Autodesk Inventor part; units mm, degrees
(part 2 of 2)
  line L274 (138.3563, 14.6531) -> (138.3563, 9.9031)
  line L275 (136.8563, 14.8531) -> (136.8563, 12.9031)
  line L276 (137.8563, 15.1531) -> (137.8563, 15.0531)
  line L277 (138.0563, 14.8531) -> (138.1563, 14.8531)
  line L278 (137.3563, 15.3531) -> (137.6563, 15.3531)
  line L279 (138.0563, 21.8531) -> (138.1563, 21.8531)
  line L280 (137.8563, 21.5531) -> (137.8563, 21.6531)
  line L281 (137.3563, 21.3531) -> (137.6563, 21.3531)
ref_plane "Start Plane" through (0, 0, 0) normal (0, 0, 1) x (1, 0, 0)
ref_plane "End Plane" through (0, 0, 150) normal (0, 0, 1) x (1, 0, 0)
sketch "Sketch1" plane through (0, 0, 0) normal (0, 0, 1) x (1, 0, 0)
  line L0 (-3.2324, -15.4999) -> (-0.9538, -15.4999)
  arc A0 (-0.8538, -15.5267) -> (-0.9538, -15.4999) centre (-0.9538, -15.6999) ccw
  line L1 (-0.8538, -15.5267) -> (-0.1, -15.9619)
  arc A1 (-0.1, -15.9619) -> (0.1, -15.9619) centre (0, -15.7887) ccw
  line L2 (0.1, -15.9619) -> (0.8538, -15.5267)
  arc A2 (0.9538, -15.4999) -> (0.8538, -15.5267) centre (0.9538, -15.6999) ccw
  line L3 (0.9538, -15.4999) -> (3.2324, -15.4999)
  arc A3 (3.2324, -15.4999) -> (3.586, -15.3534) centre (3.2324, -14.9999) ccw
  line L4 (3.586, -15.3534) -> (6.2929, -12.6465)
  arc A4 (6.6464, -12.5) -> (6.2929, -12.6465) centre (6.6464, -13) ccw
  line L5 (6.6464, -12.5) -> (8, -12.5)
  arc A5 (8, -12.5) -> (8.5, -12) centre (8, -12) ccw
  line L6 (8.5, -12) -> (8.5, -8)
  arc A6 (8.5, -8) -> (8, -7.5) centre (8, -8) ccw
  line L7 (8, -7.5) -> (6.6464, -7.5)
  arc A7 (6.2929, -7.3536) -> (6.6464, -7.5) centre (6.6464, -7) ccw
  line L8 (6.2929, -7.3536) -> (3.5858, -4.6465)
  arc A8 (3.5858, -4.6465) -> (3.2322, -4.5) centre (3.2322, -5) ccw
  line L9 (3.2322, -4.5) -> (0.9536, -4.5)
  arc A9 (0.8536, -4.4732) -> (0.9536, -4.5) centre (0.9536, -4.3) ccw
  line L10 (0.8536, -4.4732) -> (0.1, -4.0381)
  arc A10 (0.1, -4.0381) -> (-0.1, -4.0381) centre (0, -4.2113) ccw
  line L11 (-0.1, -4.0381) -> (-0.8536, -4.4732)
  arc A11 (5.8536, 6.9142) -> (6, 7.2678) centre (5.5, 7.2678) ccw
  line L12 (6, 8) -> (6, 7.2678)
  arc A12 (6, 8) -> (5.5, 8.5) centre (5.5, 8) ccw
  line L13 (3.5, 8.5) -> (5.5, 8.5)
  arc A13 (3, 9) -> (3.5, 8.5) centre (3.5, 9) ccw
  line L14 (3, 9.3) -> (3, 9)
  arc A14 (3.2, 9.5) -> (3, 9.3) centre (3.2, 9.3) ccw
  line L15 (3.3, 9.5) -> (3.2, 9.5)
  arc A15 (3.3, 9.5) -> (3.5, 9.7) centre (3.3, 9.7) ccw
  line L16 (3.5, 9.8) -> (3.5, 9.7)
  arc A16 (3.7, 10) -> (3.5, 9.8) centre (3.7, 9.8) ccw
  line L17 (8.5, 10) -> (3.7, 10)
  arc A17 (10, 8.5) -> (8.5, 10) centre (8.5, 8.5) ccw
  line L18 (10, 3.7) -> (10, 8.5)
  arc A18 (9.8, 3.5) -> (10, 3.7) centre (9.8, 3.7) ccw
  line L19 (9.7, 3.5) -> (9.8, 3.5)
  arc A19 (9.7, 3.5) -> (9.5, 3.3) centre (9.7, 3.3) ccw
  line L20 (9.5, 3.2) -> (9.5, 3.3)
  arc A20 (9.3, 3) -> (9.5, 3.2) centre (9.3, 3.2) ccw
  line L21 (9, 3) -> (9.3, 3)
  arc A21 (8.5, 3.5) -> (9, 3) centre (9, 3.5) ccw
  line L22 (8.5, 5.5) -> (8.5, 3.5)
  arc A22 (8.5, 5.5) -> (8, 6) centre (8, 5.5) ccw
  line L23 (7.2678, 6) -> (8, 6)
  arc A23 (7.2678, 6) -> (6.9142, 5.8536) centre (7.2678, 5.5) ccw
  line L24 (4.6464, 3.5858) -> (6.9142, 5.8536)
  arc A24 (4.6464, 3.5858) -> (4.5, 3.2322) centre (5, 3.2322) ccw
  line L25 (4.5, 0.9536) -> (4.5, 3.2322)
  arc A25 (4.4732, 0.8536) -> (4.5, 0.9536) centre (4.3, 0.9536) ccw
  line L26 (4.0381, 0.1) -> (4.4732, 0.8536)
  arc A26 (4.0381, 0.1) -> (4.0381, -0.1) centre (4.2113, 0) ccw
  line L27 (4.4732, -0.8536) -> (4.0381, -0.1)
  arc A27 (4.5, -0.9536) -> (4.4732, -0.8536) centre (4.3, -0.9536) ccw
  line L28 (4.5, -3.2322) -> (4.5, -0.9536)
  arc A28 (4.5, -3.2322) -> (4.6464, -3.5858) centre (5, -3.2322) ccw
  line L29 (6.9142, -5.8536) -> (4.6464, -3.5858)
  arc A29 (6.9142, -5.8536) -> (7.2678, -6) centre (7.2678, -5.5) ccw
  line L30 (8, -6) -> (7.2678, -6)
  arc A30 (8, -6) -> (8.5, -5.5) centre (8, -5.5) ccw
  line L31 (8.5, -3.5) -> (8.5, -5.5)
  arc A31 (9, -3) -> (8.5, -3.5) centre (9, -3.5) ccw
  line L32 (9.3, -3) -> (9, -3)
  arc A32 (9.5, -3.2) -> (9.3, -3) centre (9.3, -3.2) ccw
  line L33 (9.5, -3.3) -> (9.5, -3.2)
  arc A33 (9.5, -3.3) -> (9.7, -3.5) centre (9.7, -3.3) ccw
  line L34 (9.8, -3.5) -> (9.7, -3.5)
  arc A34 (10, -3.7) -> (9.8, -3.5) centre (9.8, -3.7) ccw
  line L35 (10, -16.35) -> (10, -3.7)
  arc A35 (9.8, -16.55) -> (10, -16.35) centre (9.8, -16.35) ccw
  line L36 (9.7, -16.55) -> (9.8, -16.55)
  arc A36 (9.7, -16.55) -> (9.5, -16.75) centre (9.7, -16.75) ccw
  line L37 (9.5, -16.85) -> (9.5, -16.75)
  arc A37 (9.3, -17.05) -> (9.5, -16.85) centre (9.3, -16.85) ccw
  line L38 (9, -17.05) -> (9.3, -17.05)
  arc A38 (8.5, -16.55) -> (9, -17.05) centre (9, -16.55) ccw
  line L39 (8.5, -14.5) -> (8.5, -16.55)
  arc A39 (8.5, -14.5) -> (8, -14) centre (8, -14.5) ccw
  line L40 (7.2678, -14) -> (8, -14)
  arc A40 (7.2678, -14) -> (6.9142, -14.1464) centre (7.2678, -14.5) ccw
  line L41 (4.6464, -16.4142) -> (6.9142, -14.1464)
  arc A41 (4.6464, -16.4142) -> (4.5, -16.7678) centre (5, -16.7678) ccw
  line L42 (4.5, -19.0464) -> (4.5, -16.7678)
  arc A42 (4.4732, -19.1464) -> (4.5, -19.0464) centre (4.3, -19.0464) ccw
  line L43 (4.0381, -19.9) -> (4.4732, -19.1464)
  arc A43 (4.0381, -19.9) -> (4.0381, -20.1) centre (4.2113, -20) ccw
  line L44 (4.4732, -20.8536) -> (4.0381, -20.1)
  arc A44 (4.5, -20.9536) -> (4.4732, -20.8536) centre (4.3, -20.9536) ccw
  line L45 (4.5, -23.2322) -> (4.5, -20.9536)
  arc A45 (4.5, -23.2322) -> (4.6464, -23.5858) centre (5, -23.2322) ccw
  line L46 (6.9142, -25.8536) -> (4.6464, -23.5858)
  arc A46 (6.9142, -25.8536) -> (7.2678, -26) centre (7.2678, -25.5) ccw
  line L47 (8, -26) -> (7.2678, -26)
  arc A47 (8, -26) -> (8.5, -25.5) centre (8, -25.5) ccw
  line L48 (8.5, -23.55) -> (8.5, -25.5)
  arc A48 (9, -23.05) -> (8.5, -23.55) centre (9, -23.55) ccw
  line L49 (9.3, -23.05) -> (9, -23.05)
  arc A49 (9.5, -23.25) -> (9.3, -23.05) centre (9.3, -23.25) ccw
  line L50 (9.5, -23.35) -> (9.5, -23.25)
  arc A50 (9.5, -23.35) -> (9.7, -23.55) centre (9.7, -23.35) ccw
  line L51 (9.8, -23.55) -> (9.7, -23.55)
  arc A51 (10, -23.75) -> (9.8, -23.55) centre (9.8, -23.75) ccw
  arc A52 (-0.9536, -4.5) -> (-0.8536, -4.4732) centre (-0.9536, -4.3) ccw
  line L52 (-0.9536, -4.5) -> (-3.2322, -4.5)
  arc A53 (-3.2322, -4.5) -> (-3.5858, -4.6465) centre (-3.2322, -5) ccw
  line L53 (-3.5858, -4.6465) -> (-6.2929, -7.3536)
  arc A54 (-6.6464, -7.5) -> (-6.2929, -7.3536) centre (-6.6464, -7) ccw
  line L54 (-6.6464, -7.5) -> (-8, -7.5)
  arc A55 (-8, -7.5) -> (-8.5, -8) centre (-8, -8) ccw
  line L55 (-8.5, -8) -> (-8.5, -12)
  arc A56 (-8.5, -12) -> (-8, -12.5) centre (-8, -12) ccw
  line L56 (-8, -12.5) -> (-6.6464, -12.5)
  arc A57 (-6.2929, -12.6465) -> (-6.6464, -12.5) centre (-6.6464, -13) ccw
  line L57 (-6.2929, -12.6465) -> (-3.586, -15.3534)
  arc A58 (-3.586, -15.3534) -> (-3.2324, -15.4999) centre (-3.2324, -14.9999) ccw
  arc A59 (-10, -28.5) -> (-8.5, -30) centre (-8.5, -28.5) ccw
  line L58 (-10, -23.75) -> (-10, -28.5)
  arc A60 (-9.8, -23.55) -> (-10, -23.75) centre (-9.8, -23.75) ccw
  line L59 (-9.7, -23.55) -> (-9.8, -23.55)
  arc A61 (-9.7, -23.55) -> (-9.5, -23.35) centre (-9.7, -23.35) ccw
  line L60 (-9.5, -23.25) -> (-9.5, -23.35)
  arc A62 (-9.3, -23.05) -> (-9.5, -23.25) centre (-9.3, -23.25) ccw
  line L61 (-9, -23.05) -> (-9.3, -23.05)
  arc A63 (-8.5, -23.55) -> (-9, -23.05) centre (-9, -23.55) ccw
  line L62 (-8.5, -25.5) -> (-8.5, -23.55)
  arc A64 (-8.5, -25.5) -> (-8, -26) centre (-8, -25.5) ccw
  line L63 (-7.2678, -26) -> (-8, -26)
  arc A65 (-7.2678, -26) -> (-6.9142, -25.8536) centre (-7.2678, -25.5) ccw
  line L64 (-4.6464, -23.5858) -> (-6.9142, -25.8536)
  arc A66 (-4.6464, -23.5858) -> (-4.5, -23.2322) centre (-5, -23.2322) ccw
  line L65 (-4.5, -20.9536) -> (-4.5, -23.2322)
  arc A67 (-4.4732, -20.8536) -> (-4.5, -20.9536) centre (-4.3, -20.9536) ccw
  line L66 (-4.0381, -20.1) -> (-4.4732, -20.8536)
  arc A68 (-4.0381, -20.1) -> (-4.0381, -19.9) centre (-4.2113, -20) ccw
  line L67 (-4.4732, -19.1464) -> (-4.0381, -19.9)
  arc A69 (-4.5, -19.0464) -> (-4.4732, -19.1464) centre (-4.3, -19.0464) ccw
  line L68 (-4.5, -16.7678) -> (-4.5, -19.0464)
  arc A70 (-4.5, -16.7678) -> (-4.6464, -16.4142) centre (-5, -16.7678) ccw
  line L69 (-6.9142, -14.1464) -> (-4.6464, -16.4142)
  arc A71 (-6.9142, -14.1464) -> (-7.2678, -14) centre (-7.2678, -14.5) ccw
  line L70 (-8, -14) -> (-7.2678, -14)
  arc A72 (-8, -14) -> (-8.5, -14.5) centre (-8, -14.5) ccw
  line L71 (-8.5, -16.55) -> (-8.5, -14.5)
  arc A73 (-9, -17.05) -> (-8.5, -16.55) centre (-9, -16.55) ccw
  line L72 (-9.3, -17.05) -> (-9, -17.05)
  arc A74 (-9.5, -16.85) -> (-9.3, -17.05) centre (-9.3, -16.85) ccw
  line L73 (-9.5, -16.75) -> (-9.5, -16.85)
  arc A75 (-9.5, -16.75) -> (-9.7, -16.55) centre (-9.7, -16.75) ccw
  line L74 (-9.8, -16.55) -> (-9.7, -16.55)
  arc A76 (-10, -16.35) -> (-9.8, -16.55) centre (-9.8, -16.35) ccw
  line L75 (-10, -3.7) -> (-10, -16.35)
  arc A77 (-9.8, -3.5) -> (-10, -3.7) centre (-9.8, -3.7) ccw
  line L76 (-9.7, -3.5) -> (-9.8, -3.5)
  arc A78 (-9.7, -3.5) -> (-9.5, -3.3) centre (-9.7, -3.3) ccw
  line L77 (-9.5, -3.2) -> (-9.5, -3.3)
  arc A79 (-9.3, -3) -> (-9.5, -3.2) centre (-9.3, -3.2) ccw
  line L78 (-9, -3) -> (-9.3, -3)
  arc A80 (-8.5, -3.5) -> (-9, -3) centre (-9, -3.5) ccw
  line L79 (-8.5, -5.45) -> (-8.5, -3.5)
  arc A81 (-8.5, -5.45) -> (-8, -5.95) centre (-8, -5.45) ccw
  line L80 (-7.2178, -5.95) -> (-8, -5.95)
  arc A82 (-7.2178, -5.95) -> (-6.8642, -5.8036) centre (-7.2178, -5.45) ccw
  line L81 (-4.6464, -3.5858) -> (-6.8642, -5.8036)
  arc A83 (-4.6464, -3.5858) -> (-4.5, -3.2322) centre (-5, -3.2322) ccw
  line L82 (-4.5, -0.9536) -> (-4.5, -3.2322)
  arc A84 (-4.4732, -0.8536) -> (-4.5, -0.9536) centre (-4.3, -0.9536) ccw
  line L83 (-4.0381, -0.1) -> (-4.4732, -0.8536)
  arc A85 (-4.0381, -0.1) -> (-4.0381, 0.1) centre (-4.2113, 0) ccw
  line L84 (-4.4732, 0.8536) -> (-4.0381, 0.1)
  arc A86 (-4.5, 0.9536) -> (-4.4732, 0.8536) centre (-4.3, 0.9536) ccw
  line L85 (-4.5, 3.2322) -> (-4.5, 0.9536)
  arc A87 (-4.5, 3.2322) -> (-4.6464, 3.5858) centre (-5, 3.2322) ccw
  line L86 (-6.9642, 5.9036) -> (-4.6464, 3.5858)
  arc A88 (-6.9642, 5.9036) -> (-7.3178, 6.05) centre (-7.3178, 5.55) ccw
  line L87 (-8, 6.05) -> (-7.3178, 6.05)
  arc A89 (-8, 6.05) -> (-8.5, 5.55) centre (-8, 5.55) ccw
  line L88 (-8.5, 3.5) -> (-8.5, 5.55)
  arc A90 (-9, 3) -> (-8.5, 3.5) centre (-9, 3.5) ccw
  line L89 (-9.3, 3) -> (-9, 3)
  arc A91 (-9.5, 3.2) -> (-9.3, 3) centre (-9.3, 3.2) ccw
  line L90 (-9.5, 3.3) -> (-9.5, 3.2)
  arc A92 (-9.5, 3.3) -> (-9.7, 3.5) centre (-9.7, 3.3) ccw
  line L91 (-9.8, 3.5) -> (-9.7, 3.5)
  arc A93 (-10, 3.7) -> (-9.8, 3.5) centre (-9.8, 3.7) ccw
  line L92 (-10, 8.5) -> (-10, 3.7)
  arc A94 (-8.5, 10) -> (-10, 8.5) centre (-8.5, 8.5) ccw
  line L93 (-3.7, 10) -> (-8.5, 10)
  arc A95 (-3.5, 9.8) -> (-3.7, 10) centre (-3.7, 9.8) ccw
  line L94 (-3.5, 9.7) -> (-3.5, 9.8)
  arc A96 (-3.5, 9.7) -> (-3.3, 9.5) centre (-3.3, 9.7) ccw
  line L95 (-3.2, 9.5) -> (-3.3, 9.5)
  arc A97 (-3, 9.3) -> (-3.2, 9.5) centre (-3.2, 9.3) ccw
  line L96 (-3, 9) -> (-3, 9.3)
  arc A98 (-3.5, 8.5) -> (-3, 9) centre (-3.5, 9) ccw
  line L97 (-5.5, 8.5) -> (-3.5, 8.5)
  arc A99 (-5.5, 8.5) -> (-6, 8) centre (-5.5, 8) ccw
  line L98 (-6, 7.2678) -> (-6, 8)
  arc A100 (-6, 7.2678) -> (-5.8536, 6.9142) centre (-5.5, 7.2678) ccw
  line L99 (-3.5859, 4.6465) -> (-5.8536, 6.9142)
  arc A101 (-3.5859, 4.6465) -> (-3.2323, 4.5) centre (-3.2323, 5) ccw
  line L100 (-0.9537, 4.5) -> (-3.2323, 4.5)
  arc A102 (-0.8537, 4.4733) -> (-0.9537, 4.5) centre (-0.9537, 4.3) ccw
  line L101 (-0.1, 4.0381) -> (-0.8537, 4.4733)
  arc A103 (-0.1, 4.0381) -> (0.1, 4.0381) centre (0, 4.2113) ccw
  line L102 (0.8537, 4.4733) -> (0.1, 4.0381)
  arc A104 (0.9537, 4.5) -> (0.8537, 4.4733) centre (0.9537, 4.3) ccw
  line L103 (3.2323, 4.5) -> (0.9537, 4.5)
  arc A105 (3.2323, 4.5) -> (3.5859, 4.6465) centre (3.2323, 5) ccw
  line L104 (5.8536, 6.9142) -> (3.5859, 4.6465)
  arc A106 (9.5, -23.25) -> (9.3, -23.05) centre (9.3, -23.25) ccw
  arc A107 (10, -23.75) -> (9.8, -23.55) centre (9.8, -23.75) ccw
  arc A108 (9.5, -23.35) -> (9.7, -23.55) centre (9.7, -23.35) ccw
  arc A109 (9, -23.05) -> (8.5, -23.55) centre (9, -23.55) ccw
  arc A110 (9.7, -16.55) -> (9.5, -16.75) centre (9.7, -16.75) ccw
  arc A111 (9.8, -16.55) -> (10, -16.35) centre (9.8, -16.35) ccw
  arc A112 (9.3, -17.05) -> (9.5, -16.85) centre (9.3, -16.85) ccw
  arc A113 (8.5, -16.55) -> (9, -17.05) centre (9, -16.55) ccw
  arc A114 (-9.5, -16.75) -> (-9.7, -16.55) centre (-9.7, -16.75) ccw
  arc A115 (-10, -16.35) -> (-9.8, -16.55) centre (-9.8, -16.35) ccw
  arc A116 (-9.5, -16.85) -> (-9.3, -17.05) centre (-9.3, -16.85) ccw
  arc A117 (-9, -17.05) -> (-8.5, -16.55) centre (-9, -16.55) ccw
  arc A118 (-9.7, -23.55) -> (-9.5, -23.35) centre (-9.7, -23.35) ccw
  arc A119 (-9.8, -23.55) -> (-10, -23.75) centre (-9.8, -23.75) ccw
  arc A120 (-9.3, -23.05) -> (-9.5, -23.25) centre (-9.3, -23.25) ccw
  arc A121 (-8.5, -23.55) -> (-9, -23.05) centre (-9, -23.55) ccw
  arc A122 (-3.2, -29.5) -> (-3, -29.3) centre (-3.2, -29.3) ccw
  arc A123 (-3.7, -30) -> (-3.5, -29.8) centre (-3.7, -29.8) ccw
  arc A124 (-3.3, -29.5) -> (-3.5, -29.7) centre (-3.3, -29.7) ccw
  arc A125 (-3, -29) -> (-3.5, -28.5) centre (-3.5, -29) ccw
  arc A126 (3.5, -29.7) -> (3.3, -29.5) centre (3.3, -29.7) ccw
  arc A127 (3.5, -29.8) -> (3.7, -30) centre (3.7, -29.8) ccw
  arc A128 (3, -29.3) -> (3.2, -29.5) centre (3.2, -29.3) ccw
  arc A129 (3.5, -28.5) -> (3, -29) centre (3.5, -29) ccw
  arc A130 (-9.5, 3.3) -> (-9.7, 3.5) centre (-9.7, 3.3) ccw
  arc A131 (-10, 3.7) -> (-9.8, 3.5) centre (-9.8, 3.7) ccw
  arc A132 (-9.5, 3.2) -> (-9.3, 3) centre (-9.3, 3.2) ccw
  arc A133 (-9, 3) -> (-8.5, 3.5) centre (-9, 3.5) ccw
  arc A134 (-9.7, -3.5) -> (-9.5, -3.3) centre (-9.7, -3.3) ccw
  arc A135 (-9.8, -3.5) -> (-10, -3.7) centre (-9.8, -3.7) ccw
  arc A136 (-9.3, -3) -> (-9.5, -3.2) centre (-9.3, -3.2) ccw
  arc A137 (-8.5, -3.5) -> (-9, -3) centre (-9, -3.5) ccw
  arc A138 (9.5, -3.2) -> (9.3, -3) centre (9.3, -3.2) ccw
  arc A139 (10, -3.7) -> (9.8, -3.5) centre (9.8, -3.7) ccw
  arc A140 (9.5, -3.3) -> (9.7, -3.5) centre (9.7, -3.3) ccw
  arc A141 (9, -3) -> (8.5, -3.5) centre (9, -3.5) ccw
  arc A142 (9.7, 3.5) -> (9.5, 3.3) centre (9.7, 3.3) ccw
  arc A143 (9.8, 3.5) -> (10, 3.7) centre (9.8, 3.7) ccw
  arc A144 (9.3, 3) -> (9.5, 3.2) centre (9.3, 3.2) ccw
  arc A145 (8.5, 3.5) -> (9, 3) centre (9, 3.5) ccw
  arc A146 (-3, 9.3) -> (-3.2, 9.5) centre (-3.2, 9.3) ccw
  arc A147 (-3.5, 9.8) -> (-3.7, 10) centre (-3.7, 9.8) ccw
  arc A148 (-3.5, 9.7) -> (-3.3, 9.5) centre (-3.3, 9.7) ccw
  arc A149 (-3.5, 8.5) -> (-3, 9) centre (-3.5, 9) ccw
  arc A150 (3.2, 9.5) -> (3, 9.3) centre (3.2, 9.3) ccw
  arc A151 (3.7, 10) -> (3.5, 9.8) centre (3.7, 9.8) ccw
  arc A152 (3.3, 9.5) -> (3.5, 9.7) centre (3.3, 9.7) ccw
  arc A153 (3, 9) -> (3.5, 8.5) centre (3.5, 9) ccw
  arc A154 (2.4453, -1.2582) -> (2.4453, 1.2582) centre (0, 0) ccw
  arc A155 (-1.2582, -2.4453) -> (1.2582, -2.4453) centre (0, 0) ccw
  arc A156 (-2.4453, 1.2582) -> (-2.4453, -1.2582) centre (0, 0) ccw
  arc A157 (1.8871, -2.9477) -> (2.9477, -1.8871) centre (0, 0) ccw
  arc A158 (-2.9477, -1.8871) -> (-1.8871, -2.9477) centre (0, 0) ccw
  arc A159 (-1.8871, 2.9477) -> (-2.9477, 1.8871) centre (0, 0) ccw
  arc A160 (2.9477, 1.8871) -> (1.8871, 2.9477) centre (0, 0) ccw
  arc A161 (4.0381, 0.1) -> (4.0381, -0.1) centre (4.2113, 0) ccw
  arc A162 (4.5, -0.9536) -> (4.4732, -0.8536) centre (4.3, -0.9536) ccw
  arc A163 (4.4732, 0.8536) -> (4.5, 0.9536) centre (4.3, 0.9536) ccw
  arc A164 (6.9142, -5.8536) -> (7.2678, -6) centre (7.2678, -5.5) ccw
  arc A165 (4.5, -3.2322) -> (4.6464, -3.5858) centre (5, -3.2322) ccw
  arc A166 (4.6464, 3.5858) -> (4.5, 3.2322) centre (5, 3.2322) ccw
  arc A167 (7.2678, 6) -> (6.9142, 5.8536) centre (7.2678, 5.5) ccw
  arc A168 (0.1, -4.0381) -> (-0.1, -4.0381) centre (0, -4.2113) ccw
  arc A169 (-0.9536, -4.5) -> (-0.8536, -4.4732) centre (-0.9536, -4.3) ccw
  line L105 (-0.8538, -15.5267) -> (-0.1, -15.9619)
  line L106 (0.8538, -15.5267) -> (0.1, -15.9619)
  line L107 (3.2324, -15.4999) -> (0.9538, -15.4999)
  line L108 (4.6464, -16.4142) -> (6.9142, -14.1464)
  line L109 (2.4453, -21.2582) -> (2.9477, -21.8871)
  line L110 (7.2678, -14) -> (8, -14)
  line L111 (7.2678, -26) -> (8, -26)
  line L112 (4.5, -16.7678) -> (4.5, -19.0464)
  line L113 (4.4732, -19.1464) -> (4.0381, -19.9)
  line L114 (4.4732, -20.8536) -> (4.0381, -20.1)
  line L115 (4.5, -23.2322) -> (4.5, -20.9536)
  line L116 (4.6464, -23.5858) -> (6.9142, -25.8536)
  line L117 (3.5858, -24.6464) -> (5.8536, -26.9142)
  line L118 (-1.2582, -22.4453) -> (-1.8871, -22.9477)
  line L119 (-2.4453, -21.2582) -> (-2.9477, -21.8871)
  line L120 (-2.4453, -18.7418) -> (-2.9477, -18.1129)
  line L121 (-1.2582, -17.5547) -> (-1.8871, -17.0523)
  line L122 (1.2582, -17.5547) -> (1.8871, -17.0523)
  line L123 (2.4453, -18.7418) -> (2.9477, -18.1129)
  line L124 (6.6464, -7.5) -> (8, -7.5)
  line L125 (8.5, -12) -> (8.5, -8)
  line L126 (6.6464, -12.5) -> (8, -12.5)
  line L127 (-6.6464, -12.5) -> (-8, -12.5)
  line L128 (-8.5, -12) -> (-8.5, -8)
  line L129 (-6.6464, -7.5) -> (-8, -7.5)
  arc A170 (1.8871, -22.9477) -> (2.9477, -21.8871) centre (0, -20) ccw
  line L130 (2.9477, -21.8871) -> (2.4453, -21.2582)
  arc A171 (2.4453, -21.2582) -> (2.4453, -18.7418) centre (0, -20) ccw
  line L131 (2.4453, -18.7418) -> (2.9477, -18.1129)
  arc A172 (2.9477, -18.1129) -> (1.8871, -17.0523) centre (0, -20) ccw
  line L132 (1.8871, -17.0523) -> (1.2582, -17.5547)
  arc A173 (1.2582, -17.5547) -> (-1.2582, -17.5547) centre (0, -20) ccw
  line L133 (-1.2582, -17.5547) -> (-1.8871, -17.0523)
  arc A174 (-1.8871, -17.0523) -> (-2.9477, -18.1129) centre (0, -20) ccw
  line L134 (-2.9477, -18.1129) -> (-2.4453, -18.7418)
  arc A175 (-2.4453, -18.7418) -> (-2.4453, -21.2582) centre (0, -20) ccw
  line L135 (-2.4453, -21.2582) -> (-2.9477, -21.8871)
  arc A176 (-2.9477, -21.8871) -> (-1.8871, -22.9477) centre (0, -20) ccw
  line L136 (-1.8871, -22.9477) -> (-1.2582, -22.4453)
  arc A177 (-1.2582, -22.4453) -> (1.2582, -22.4453) centre (0, -20) ccw
  line L137 (1.2582, -22.4453) -> (1.8871, -22.9477)
  arc A178 (2.9477, 1.8871) -> (1.8871, 2.9477) centre (0, 0) ccw
  line L138 (1.8871, 2.9477) -> (1.2582, 2.4453)
  arc A179 (1.2582, 2.4453) -> (-1.2582, 2.4453) centre (0, 0) ccw
  line L139 (-1.2582, 2.4453) -> (-1.8871, 2.9477)
  arc A180 (-1.8871, 2.9477) -> (-2.9477, 1.8871) centre (0, 0) ccw
  line L140 (-2.9477, 1.8871) -> (-2.4453, 1.2582)
  arc A181 (-2.4453, 1.2582) -> (-2.4453, -1.2582) centre (0, 0) ccw
  line L141 (-2.4453, -1.2582) -> (-2.9477, -1.8871)
  arc A182 (-2.9477, -1.8871) -> (-1.8871, -2.9477) centre (0, 0) ccw
  line L142 (-1.8871, -2.9477) -> (-1.2582, -2.4453)
  arc A183 (-1.2582, -2.4453) -> (1.2582, -2.4453) centre (0, 0) ccw
  line L143 (1.2582, -2.4453) -> (1.8871, -2.9477)
  arc A184 (1.8871, -2.9477) -> (2.9477, -1.8871) centre (0, 0) ccw
  line L144 (2.9477, -1.8871) -> (2.4453, -1.2582)
  arc A185 (2.4453, -1.2582) -> (2.4453, 1.2582) centre (0, 0) ccw
  line L145 (2.4453, 1.2582) -> (2.9477, 1.8871)
  line L146 (10, -28.5) -> (10, -23.75)
  arc A186 (8.5, -30) -> (10, -28.5) centre (8.5, -28.5) ccw
  line L147 (3.7, -30) -> (8.5, -30)
  arc A187 (3.5, -29.8) -> (3.7, -30) centre (3.7, -29.8) ccw
  line L148 (3.5, -29.7) -> (3.5, -29.8)
  arc A188 (3.5, -29.7) -> (3.3, -29.5) centre (3.3, -29.7) ccw
  line L149 (3.2, -29.5) -> (3.3, -29.5)
  arc A189 (3, -29.3) -> (3.2, -29.5) centre (3.2, -29.3) ccw
  line L150 (3, -29) -> (3, -29.3)
  arc A190 (3.5, -28.5) -> (3, -29) centre (3.5, -29) ccw
  line L151 (5.5, -28.5) -> (3.5, -28.5)
  arc A191 (5.5, -28.5) -> (6, -28) centre (5.5, -28) ccw
  line L152 (6, -27.2678) -> (6, -28)
  arc A192 (6, -27.2678) -> (5.8536, -26.9142) centre (5.5, -27.2678) ccw
  line L153 (3.5858, -24.6464) -> (5.8536, -26.9142)
  arc A193 (3.5858, -24.6464) -> (3.2322, -24.5) centre (3.2322, -25) ccw
  line L154 (0.9536, -24.5) -> (3.2322, -24.5)
  arc A194 (0.8536, -24.4732) -> (0.9536, -24.5) centre (0.9536, -24.3) ccw
  line L155 (0.1, -24.0381) -> (0.8536, -24.4732)
  arc A195 (0.1, -24.0381) -> (-0.1, -24.0381) centre (0, -24.2113) ccw
  line L156 (-0.8536, -24.4732) -> (-0.1, -24.0381)
  arc A196 (-0.9536, -24.5) -> (-0.8536, -24.4732) centre (-0.9536, -24.3) ccw
  line L157 (-3.2322, -24.5) -> (-0.9536, -24.5)
  arc A197 (-3.2322, -24.5) -> (-3.5858, -24.6464) centre (-3.2322, -25) ccw
  line L158 (-5.8536, -26.9142) -> (-3.5858, -24.6464)
  arc A198 (-5.8536, -26.9142) -> (-6, -27.2678) centre (-5.5, -27.2678) ccw
  line L159 (-6, -28) -> (-6, -27.2678)
  arc A199 (-6, -28) -> (-5.5, -28.5) centre (-5.5, -28) ccw
  line L160 (-3.5, -28.5) -> (-5.5, -28.5)
  arc A200 (-3, -29) -> (-3.5, -28.5) centre (-3.5, -29) ccw
  line L161 (-3, -29.3) -> (-3, -29)
  arc A201 (-3.2, -29.5) -> (-3, -29.3) centre (-3.2, -29.3) ccw
  line L162 (-3.3, -29.5) -> (-3.2, -29.5)
  arc A202 (-3.3, -29.5) -> (-3.5, -29.7) centre (-3.3, -29.7) ccw
  line L163 (-3.5, -29.8) -> (-3.5, -29.7)
  arc A203 (-3.7, -30) -> (-3.5, -29.8) centre (-3.7, -29.8) ccw
  line L164 (-8.5, -30) -> (-3.7, -30)
  line L165 (8.5, -16.55) -> (8.5, -14.5)
  line L166 (10, -16.35) -> (10, -10)
  line L167 (-9.7, -16.55) -> (-9.8, -16.55)
  line L168 (-9.5, -16.85) -> (-9.5, -16.75)
  line L169 (-9, -17.05) -> (-9.3, -17.05)
  line L170 (-8.5, -16.55) -> (-8.5, -14.5)
  line L171 (-10, -16.35) -> (-10, -10)
  line L172 (-9.7, -23.55) -> (-9.8, -23.55)
  line L173 (-9.5, -23.25) -> (-9.5, -23.35)
  line L174 (-9, -23.05) -> (-9.3, -23.05)
  line L175 (-8.5, -23.55) -> (-8.5, -25.5)
  line L176 (-10, -23.75) -> (-10, -28.5)
  line L177 (-3.7, -30) -> (-8.5, -30)
  line L178 (-3.5, -28.5) -> (-5.5, -28.5)
  line L179 (-3.2, -29.5) -> (-3.3, -29.5)
  line L180 (-3.5, -29.7) -> (-3.5, -29.8)
  line L181 (-3, -29) -> (-3, -29.3)
  line L182 (3.7, -30) -> (8.5, -30)
  line L183 (3.5, -29.7) -> (3.5, -29.8)
  line L184 (3.2, -29.5) -> (3.3, -29.5)
  line L185 (3, -29) -> (3, -29.3)
  line L186 (3.5, -28.5) -> (5.5, -28.5)
  line L187 (-9.7, 3.5) -> (-9.8, 3.5)
  line L188 (-9.5, 3.2) -> (-9.5, 3.3)
  line L189 (-9, 3) -> (-9.3, 3)
  line L190 (-8.5, 3.5) -> (-8.5, 5.55)
  line L191 (-10, 3.7) -> (-10, 8.5)
  line L192 (-9.7, -3.5) -> (-9.8, -3.5)
  line L193 (-9.5, -3.2) -> (-9.5, -3.3)
  line L194 (-9, -3) -> (-9.3, -3)
  line L195 (-8.5, -3.5) -> (-8.5, -5.45)
  line L196 (-10, -3.7) -> (-10, -10)
  line L197 (10, -3.7) -> (10, -10)
  line L198 (8.5, -3.5) -> (8.5, -5.5)
  line L199 (9.5, -3.2) -> (9.5, -3.3)
  line L200 (9.7, -3.5) -> (9.8, -3.5)
  line L201 (9, -3) -> (9.3, -3)
  line L202 (9.7, 3.5) -> (9.8, 3.5)
  line L203 (9.5, 3.2) -> (9.5, 3.3)
  line L204 (9, 3) -> (9.3, 3)
  line L205 (8.5, 3.5) -> (8.5, 5.5)
  line L206 (10, 3.7) -> (10, 8.5)
  line L207 (-3.7, 10) -> (-8.5, 10)
  line L208 (-3.5, 8.5) -> (-5.5, 8.5)
  line L209 (-3, 9) -> (-3, 9.3)
  line L210 (-3.2, 9.5) -> (-3.3, 9.5)
  line L211 (-3.5, 9.7) -> (-3.5, 9.8)
  line L212 (3.7, 10) -> (8.5, 10)
  line L213 (3.5, 8.5) -> (5.5, 8.5)
  line L214 (3.2, 9.5) -> (3.3, 9.5)
  line L215 (3.5, 9.7) -> (3.5, 9.8)
  line L216 (3, 9) -> (3, 9.3)
  line L217 (2.4453, -1.2582) -> (2.9477, -1.8871)
  line L218 (1.2582, -2.4453) -> (1.8871, -2.9477)
  line L219 (-1.2582, -2.4453) -> (-1.8871, -2.9477)
  line L220 (-2.4453, -1.2582) -> (-2.9477, -1.8871)
  line L221 (-2.4453, 1.2582) -> (-2.9477, 1.8871)
  line L222 (-1.2582, 2.4453) -> (-1.8871, 2.9477)
  line L223 (3.5859, 4.6465) -> (5.8536, 6.9142)
  line L224 (4.6464, 3.5858) -> (6.9142, 5.8536)
  line L225 (4.5, 3.2322) -> (4.5, 0.9536)
  line L226 (4.4732, 0.8536) -> (4.0381, 0.1)
  line L227 (4.4732, -0.8536) -> (4.0381, -0.1)
  line L228 (4.5, -3.2322) -> (4.5, -0.9536)
  line L229 (7.2678, 6) -> (8, 6)
  line L230 (7.2678, -6) -> (8, -6)
  line L231 (2.4453, 1.2582) -> (2.9477, 1.8871)
  line L232 (4.6464, -3.5858) -> (6.9142, -5.8536)
  line L233 (3.2322, -4.5) -> (0.9536, -4.5)
  line L234 (0.8536, -4.4732) -> (0.1, -4.0381)
  line L235 (-0.8536, -4.4732) -> (-0.1, -4.0381)
  line L236 (-3.2322, -4.5) -> (-0.9536, -4.5)
  line L237 (3.5858, -4.6465) -> (6.2929, -7.3536)
  line L238 (-3.5858, -4.6465) -> (-6.2929, -7.3536)
  line L239 (-4.5, -3.2322) -> (-4.5, -0.9536)
  line L240 (-4.4732, -0.8536) -> (-4.0381, -0.1)
  line L241 (-4.4732, 0.8536) -> (-4.0381, 0.1)
  line L242 (-4.5, 3.2322) -> (-4.5, 0.9536)
  line L243 (-7.2178, -5.95) -> (-8, -5.95)
  line L244 (-7.3178, 6.05) -> (-8, 6.05)
  line L245 (-4.6464, -3.5858) -> (-6.8642, -5.8036)
  line L246 (-4.6464, 3.5858) -> (-6.9642, 5.9036)
  line L247 (1.2582, 2.4453) -> (1.8871, 2.9477)
  line L248 (-3.5859, 4.6465) -> (-5.8536, 6.9142)
  line L249 (6, 7.2678) -> (6, 8)
  line L250 (-6, 7.2678) -> (-6, 8)
  line L251 (3.2323, 4.5) -> (0.9537, 4.5)
  line L252 (0.8537, 4.4733) -> (0.1, 4.0381)
  line L253 (-0.8537, 4.4733) -> (-0.1, 4.0381)
  line L254 (-3.2323, 4.5) -> (-0.9537, 4.5)
  line L255 (-3.2322, -24.5) -> (-0.9536, -24.5)
  line L256 (-0.8536, -24.4732) -> (-0.1, -24.0381)
  line L257 (0.8536, -24.4732) -> (0.1, -24.0381)
  line L258 (3.2322, -24.5) -> (0.9536, -24.5)
  line L259 (-6, -27.2678) -> (-6, -28)
  line L260 (6, -27.2678) -> (6, -28)
  line L261 (-3.5858, -24.6464) -> (-5.8536, -26.9142)
  line L262 (1.2582, -22.4453) -> (1.8871, -22.9477)
  line L263 (-4.6464, -23.5858) -> (-6.9142, -25.8536)
  line L264 (-4.6464, -16.4142) -> (-6.9142, -14.1464)
  line L265 (-7.2678, -26) -> (-8, -26)
  line L266 (-7.2678, -14) -> (-8, -14)
  line L267 (-4.5, -23.2322) -> (-4.5, -20.9536)
  line L268 (-4.4732, -20.8536) -> (-4.0381, -20.1)
  line L269 (-4.4732, -19.1464) -> (-4.0381, -19.9)
  line L270 (-4.5, -16.7678) -> (-4.5, -19.0464)
  line L271 (-3.586, -15.3534) -> (-6.2929, -12.6465)
  line L272 (3.586, -15.3534) -> (6.2929, -12.6465)
  line L273 (-3.2324, -15.4999) -> (-0.9538, -15.4999)
  arc A204 (0.8536, -4.4732) -> (0.9536, -4.5) centre (0.9536, -4.3) ccw
  arc A205 (-3.2322, -4.5) -> (-3.5858, -4.6465) centre (-3.2322, -5) ccw
  arc A206 (3.5858, -4.6465) -> (3.2322, -4.5) centre (3.2322, -5) ccw
  arc A207 (-4.0381, -0.1) -> (-4.0381, 0.1) centre (-4.2113, 0) ccw
  arc A208 (-4.5, 0.9536) -> (-4.4732, 0.8536) centre (-4.3, 0.9536) ccw
  arc A209 (-4.4732, -0.8536) -> (-4.5, -0.9536) centre (-4.3, -0.9536) ccw
  arc A210 (-6.9642, 5.9036) -> (-7.3178, 6.05) centre (-7.3178, 5.55) ccw
  arc A211 (-4.5, 3.2322) -> (-4.6464, 3.5858) centre (-5, 3.2322) ccw
  arc A212 (-4.6464, -3.5858) -> (-4.5, -3.2322) centre (-5, -3.2322) ccw
  arc A213 (-7.2178, -5.95) -> (-6.8642, -5.8036) centre (-7.2178, -5.45) ccw
  arc A214 (-6, 7.2678) -> (-5.8536, 6.9142) centre (-5.5, 7.2678) ccw
  arc A215 (-3.5859, 4.6465) -> (-3.2323, 4.5) centre (-3.2323, 5) ccw
  arc A216 (3.2323, 4.5) -> (3.5859, 4.6465) centre (3.2323, 5) ccw
  arc A217 (5.8536, 6.9142) -> (6, 7.2678) centre (5.5, 7.2678) ccw
  arc A218 (8.5, 5.5) -> (8, 6) centre (8, 5.5) ccw
  arc A219 (10, 8.5) -> (8.5, 10) centre (8.5, 8.5) ccw
  arc A220 (8, -6) -> (8.5, -5.5) centre (8, -5.5) ccw
  arc A221 (-8.5, -5.45) -> (-8, -5.95) centre (-8, -5.45) ccw
  arc A222 (-8, 6.05) -> (-8.5, 5.55) centre (-8, 5.55) ccw
  arc A223 (6, 8) -> (5.5, 8.5) centre (5.5, 8) ccw
  arc A224 (-8.5, 10) -> (-10, 8.5) centre (-8.5, 8.5) ccw
  arc A225 (-5.5, 8.5) -> (-6, 8) centre (-5.5, 8) ccw
  arc A226 (-0.8537, 4.4733) -> (-0.9537, 4.5) centre (-0.9537, 4.3) ccw
  arc A227 (0.9537, 4.5) -> (0.8537, 4.4733) centre (0.9537, 4.3) ccw
  arc A228 (-0.1, 4.0381) -> (0.1, 4.0381) centre (0, 4.2113) ccw
  arc A229 (1.2582, 2.4453) -> (-1.2582, 2.4453) centre (0, 0) ccw
  arc A230 (-1.2582, -22.4453) -> (1.2582, -22.4453) centre (0, -20) ccw
  arc A231 (0.1, -24.0381) -> (-0.1, -24.0381) centre (0, -24.2113) ccw
  arc A232 (0.8536, -24.4732) -> (0.9536, -24.5) centre (0.9536, -24.3) ccw
  arc A233 (-0.9536, -24.5) -> (-0.8536, -24.4732) centre (-0.9536, -24.3) ccw
  arc A234 (-6, -28) -> (-5.5, -28.5) centre (-5.5, -28) ccw
  arc A235 (-10, -28.5) -> (-8.5, -30) centre (-8.5, -28.5) ccw
  arc A236 (5.5, -28.5) -> (6, -28) centre (5.5, -28) ccw
  arc A237 (-8.5, -25.5) -> (-8, -26) centre (-8, -25.5) ccw
  arc A238 (-8, -14) -> (-8.5, -14.5) centre (-8, -14.5) ccw
  arc A239 (8.5, -14.5) -> (8, -14) centre (8, -14.5) ccw
  arc A240 (8.5, -30) -> (10, -28.5) centre (8.5, -28.5) ccw
  arc A241 (8, -26) -> (8.5, -25.5) centre (8, -25.5) ccw
  arc A242 (6, -27.2678) -> (5.8536, -26.9142) centre (5.5, -27.2678) ccw
  arc A243 (3.5858, -24.6464) -> (3.2322, -24.5) centre (3.2322, -25) ccw
  arc A244 (-3.2322, -24.5) -> (-3.5858, -24.6464) centre (-3.2322, -25) ccw
  arc A245 (-5.8536, -26.9142) -> (-6, -27.2678) centre (-5.5, -27.2678) ccw
  arc A246 (-6.9142, -14.1464) -> (-7.2678, -14) centre (-7.2678, -14.5) ccw
  arc A247 (-4.5, -16.7678) -> (-4.6464, -16.4142) centre (-5, -16.7678) ccw
  arc A248 (-4.6464, -23.5858) -> (-4.5, -23.2322) centre (-5, -23.2322) ccw
  arc A249 (-7.2678, -26) -> (-6.9142, -25.8536) centre (-7.2678, -25.5) ccw
  arc A250 (-4.5, -19.0464) -> (-4.4732, -19.1464) centre (-4.3, -19.0464) ccw
  arc A251 (-4.4732, -20.8536) -> (-4.5, -20.9536) centre (-4.3, -20.9536) ccw
  arc A252 (-4.0381, -20.1) -> (-4.0381, -19.9) centre (-4.2113, -20) ccw
  arc A253 (3.2324, -15.4999) -> (3.586, -15.3534) centre (3.2324, -14.9999) ccw
  arc A254 (-3.586, -15.3534) -> (-3.2324, -15.4999) centre (-3.2324, -14.9999) ccw
  arc A255 (0.9538, -15.4999) -> (0.8538, -15.5267) centre (0.9538, -15.6999) ccw
  arc A256 (-0.8538, -15.5267) -> (-0.9538, -15.4999) centre (-0.9538, -15.6999) ccw
  arc A257 (-0.1, -15.9619) -> (0.1, -15.9619) centre (0, -15.7887) ccw
  arc A258 (6.9142, -25.8536) -> (7.2678, -26) centre (7.2678, -25.5) ccw
  arc A259 (4.5, -23.2322) -> (4.6464, -23.5858) centre (5, -23.2322) ccw
  arc A260 (4.6464, -16.4142) -> (4.5, -16.7678) centre (5, -16.7678) ccw
  arc A261 (7.2678, -14) -> (6.9142, -14.1464) centre (7.2678, -14.5) ccw
  arc A262 (4.5, -20.9536) -> (4.4732, -20.8536) centre (4.3, -20.9536) ccw
  arc A263 (4.4732, -19.1464) -> (4.5, -19.0464) centre (4.3, -19.0464) ccw
  arc A264 (4.0381, -19.9) -> (4.0381, -20.1) centre (4.2113, -20) ccw
  arc A265 (1.8871, -22.9477) -> (2.9477, -21.8871) centre (0, -20) ccw
  arc A266 (-2.9477, -21.8871) -> (-1.8871, -22.9477) centre (0, -20) ccw
  arc A267 (-1.8871, -17.0523) -> (-2.9477, -18.1129) centre (0, -20) ccw
  arc A268 (2.9477, -18.1129) -> (1.8871, -17.0523) centre (0, -20) ccw
  arc A269 (-2.4453, -18.7418) -> (-2.4453, -21.2582) centre (0, -20) ccw
  arc A270 (1.2582, -17.5547) -> (-1.2582, -17.5547) centre (0, -20) ccw
  arc A271 (2.4453, -21.2582) -> (2.4453, -18.7418) centre (0, -20) ccw
  arc A272 (-6.6464, -7.5) -> (-6.2929, -7.3536) centre (-6.6464, -7) ccw
  arc A273 (-8, -7.5) -> (-8.5, -8) centre (-8, -8) ccw
  arc A274 (-8.5, -12) -> (-8, -12.5) centre (-8, -12) ccw
  arc A275 (-6.2929, -12.6465) -> (-6.6464, -12.5) centre (-6.6464, -13) ccw
  arc A276 (6.2929, -7.3536) -> (6.6464, -7.5) centre (6.6464, -7) ccw
  arc A277 (8.5, -8) -> (8, -7.5) centre (8, -8) ccw
  arc A278 (8, -12.5) -> (8.5, -12) centre (8, -12) ccw
  arc A279 (6.6464, -12.5) -> (6.2929, -12.6465) centre (6.6464, -13) ccw
  line L274 (10, -23.75) -> (10, -28.5)
  line L275 (8.5, -23.55) -> (8.5, -25.5)
  line L276 (9.5, -23.25) -> (9.5, -23.35)
  line L277 (9.7, -23.55) -> (9.8, -23.55)
  line L278 (9, -23.05) -> (9.3, -23.05)
  line L279 (9.7, -16.55) -> (9.8, -16.55)
  line L280 (9.5, -16.85) -> (9.5, -16.75)
  line L281 (9, -17.05) -> (9.3, -17.05)
  constraints: 1 other
extrude "Body" add sketch "Sketch1" along normal up to surface (150 mm away) from surface at 0
sketch "Sketch10" plane through (0, 0, 0) normal (0, 0, 1) x (1, 0, 0)
  line L0 (0, 0) -> (10, 0)
ref_plane "Work Plane9" through (0, 0, 0) normal (0, -1, 0) x (1, 0, 0)
sketch "Sketch11" plane through (0, 0, 0) normal (0, -1, 0) x (1, 0, 0)
  line L0 (-2, 0) -> (12, 0)
  line L1 (-2, 150) -> (12, 150)
  dimension "d21" = 150
  measures "d21" distance between parallel lines of L0 L1
sketch "Sketch12" plane through (10, -16.35, 150) normal (1, 0, 0) x (0, 0, -1)
  circle A0 centre (267.0792, -35.2322) radius 2.55 projected
  circle A1 centre (287.0792, -35.2322) radius 2.55 projected
  point P0 (150, 16.35)
  constraints: 2 coincident
hole "Hole1" at (10, -51.5822, -117.0792) at (10, -51.5822, -137.0792) direction (-1, 0, 0) diameter 5.1 end through all
equation "\"G_OFFSET_START\" = 0"
equation "\"G_OFFSET_END\" = 0"
equation "\"G_L\" = d21"
body "Solid2"
